Rondelle suspension (Autodesk Fusion 360 design; units mm, degrees)
Autodesk Fusion 360 part; units mm, degrees
sketch "Sketch1" plane through (0, 0, 0) normal (0, 0, 1) x (1, 0, 0)
  line L0 (-7.5026, 28) -> (-20.4974, 20.4974)
  line L1 (-20.4974, 20.4974) -> (-28, 7.5026)
  line L2 (-28, 7.5026) -> (-28, -7.5026)
  line L3 (-28, -7.5026) -> (-20.4974, -20.4974)
  line L4 (-20.4974, -20.4974) -> (-7.5026, -28)
  line L5 (-7.5026, -28) -> (7.5026, -28)
  line L6 (7.5026, -28) -> (20.4974, -20.4974)
  line L7 (20.4974, -20.4974) -> (28, -7.5026)
  line L8 (28, -7.5026) -> (28, 7.5026)
  line L9 (28, 7.5026) -> (20.4974, 20.4974)
  line L10 (20.4974, 20.4974) -> (7.5026, 28)
  line L11 (7.5026, 28) -> (-7.5026, 28)
  circle A0 centre (0, 0) radius 22.5 construction
  line L12 (0, 0) -> (0, 28) construction
  circle A1 centre (0, 22.5) radius 2.1
  circle A2 centre (-19.4856, 11.25) radius 2.1
  circle A3 centre (-19.4856, -11.25) radius 2.1
  circle A4 centre (0, -22.5) radius 2.1
  circle A5 centre (19.4856, -11.25) radius 2.1
  circle A6 centre (19.4856, 11.25) radius 2.1
  circle A7 centre (0, 0) radius 15
  dimension "d1" = 28
  dimension "d2" = 45
  dimension "d3" = 4.2
  dimension "d5" = 360
  dimension "d6" = 30
  constraint coincident A0.centre L12.start
  constraint midpoint L11 L12.end
  constraint coincident A0 A1.centre
  constraint coincident L12 A1.centre
  constraint concentric A0 A7
  measures "d1" distance of A0.centre L11
  measures "d2" diameter of A0
  measures "d3" diameter of A1
  measures "d6" diameter of A7
extrude "Extrude1" add sketch "Sketch1" along normal blind 2
